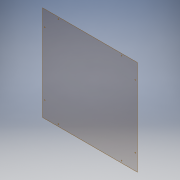
# Autodesk Inventor part: Fundo Gaveta
Saved by Autodesk Inventor 2018 (Build 220112000, 112)
## iProperties
Created: 2018-07-08
Part Number: Fundo Gaveta
Material: PMMA plástico
Document SubType Name: Chapa de metal
Designer: Regner
Density: 1.188 g/cm^3
Sheet Metal Rule: Padrão_mm
Appearance: Policarbonato - Fumê
Author: Regner
Autodesk Inventor part; units mm, degrees
ref_plane "YZ Plane" through (0, 0, 0) normal (1, 0, 0) x (0, 1, 0)
ref_plane "XZ Plane" through (0, 0, 0) normal (0, 1, 0) x (-1, 0, 0)
ref_plane "XY Plane" through (0, 0, 0) normal (0, 0, 1) x (1, 0, 0)
sketch "Esboço1" plane through (0, 0, 0) normal (0, 1, 0) x (-1, 0, 0)
  line L0 (-149, -149) -> (149, -149)
  line L1 (149, -149) -> (149, 149)
  line L2 (149, 149) -> (-149, 149)
  line L3 (-149, 149) -> (-149, -149)
  line L4 (-149, -149) -> (149, 149) construction
  line L5 (149, -149) -> (-149, 149) construction
  point P0 (0, 0)
  dimension "d0" = 298
  dimension "d1" = 298
  measures "d0" distance of L2.end L1.end
  measures "d1" distance of L2.end L0.start
extrude "Placa1" add sketch "Esboço1" along normal blind 0.5
sketch "Esboço2" plane through (0, 0, 0) normal (0, -1, 0) x (1, 0, 0)
  line L0 (-149, 149) -> (149, 149) projected
  line L1 (149, -149) -> (-149, -149) projected
  line L2 (-149, -149) -> (-149, 149) projected
  line L3 (149, 149) -> (149, -149) projected
  point P0 (0, 0)
  point P1 (-99, 143)
  point P2 (99, 143)
  point P3 (142.5, 99)
  point P4 (142.5, -99)
  point P5 (99, -142.5)
  point P6 (-99, -142.5)
  point P7 (-142.5, -99)
  point P8 (-142.5, 99)
  dimension "d3" = 50
  dimension "d4" = 50
  dimension "d5" = 50
  dimension "d6" = 50
  dimension "d7" = 50
  dimension "d8" = 50
  dimension "d9" = 50
  dimension "d10" = 50
  dimension "d11" = 6
  dimension "d12" = 6
  dimension "d13" = 6.5
  dimension "d14" = 6.5
  dimension "d15" = 6.5
  dimension "d16" = 6.5
  dimension "d17" = 6.5
  dimension "d18" = 6.5
  measures "d3" distance from line of L0 point (-142.5, 99)
  measures "d4" distance from line of L1 point (-142.5, -99)
  measures "d5" distance from line of L2 point (-99, -142.5)
  measures "d6" distance from line of L3 point (99, -142.5)
  measures "d7" distance from line of L1 point (142.5, -99)
  measures "d8" distance from line of L0 point (142.5, 99)
  measures "d9" distance from line of L3 point (99, 143)
  measures "d10" distance from line of L2 point (-99, 143)
  measures "d11" distance from line of L0 point (-99, 143)
  measures "d12" distance from line of L0 point (99, 143)
  measures "d13" distance from line of L3 point (142.5, 99)
  measures "d14" distance from line of L2 point (-142.5, 99)
  measures "d15" distance from line of L2 point (-142.5, -99)
  measures "d16" distance from line of L3 point (142.5, -99)
  measures "d17" distance from line of L1 point (99, -142.5)
  measures "d18" distance from line of L1 point (-99, -142.5)
hole "Furo1" at (-99, 0, 143) at (99, 0, 143) at (142.5, 0, 99) at (142.5, 0, -99) at (99, 0, -142.5) at (-99, 0, -142.5) at (-142.5, 0, -99) at (-142.5, 0, 99) direction (0, 1, 0) diameter 3 end through all
equation "\"d1\" = d0"
equation "\"d24\" = Espessura"
equation "\"d2\" = Espessura"
equation "\"Raio_vergadura\" = Espessura"
equation "\"Largura_alívio_de_vergadura\" = Espessura"
equation "\"Profundidade_alívio_de_vergadura\" = 0.5 * Espessura"
equation "\"Tamanho_alívio_de_dobra\" = 4 * Espessura"
equation "\"Remanescente_mínimo\" = 2 * Espessura"
equation "\"Raiodetransição\" = Raio_vergadura"
equation "\"Tamanho_de_raio_de_Jacobi\" = Raio_vergadura"
equation "\"TamanhoFolga\" = Espessura"
equation "\"Espessura\" = 0.5"
